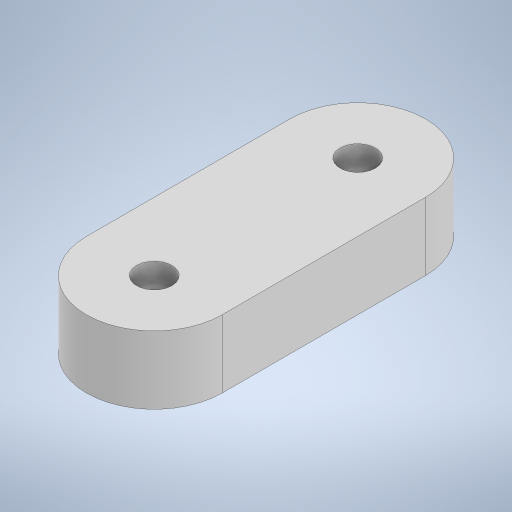
# Autodesk Inventor part: Zarmattacher
Saved by Autodesk Inventor 2023 (Build 270158000, 158)
## iProperties
Created: 2023-10-26
Part Number: Zarmattacher
Material: Generic
Document SubType Name: Modeling
Designer: Mustapha
Density: 1 g/cm^3
Appearance: Default
Author: Mustapha
Autodesk Inventor part; units mm, degrees
ref_plane "YZ Plane" through (0, 0, 0) normal (1, 0, 0) x (0, 1, 0)
ref_plane "XZ Plane" through (0, 0, 0) normal (0, 1, 0) x (-1, 0, 0)
ref_plane "XY Plane" through (0, 0, 0) normal (0, 0, 1) x (1, 0, 0)
sketch "Sketch1" plane through (0, 0, 0) normal (0, 1, 0) x (-1, 0, 0)
  line L0 (0, 15) -> (0, -15) construction
  line L1 (-10, 15) -> (-10, -15)
  line L2 (10, -15) -> (10, 15)
  arc A0 (10, 15) -> (-10, 15) centre (0, 15) ccw
  arc A1 (-10, -15) -> (10, -15) centre (0, -15) ccw
  circle A2 centre (0, -15) radius 2.6
  circle A3 centre (0, 15) radius 2.6
  point P0 (0, 0)
  dimension "d0" = 5.2
  dimension "d1" = 5.2
  dimension "d2" = 30
  dimension "d3" = 20
  constraints: 8 end point, 4 centre point, 4 point on circle, 4 tangent, 2 coincident, 1 midpoint, 1 parallel, 1 vertical
  measures "d0" diameter of A3
  measures "d1" diameter of A2
  measures "d2" distance of L0.end L0.start
  measures "d3" distance between parallel lines of L1 L2
extrude "Extrusion1" add sketch "Sketch1" along normal blind 10
body "Solid1"
